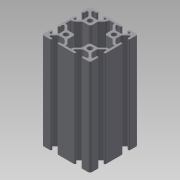
# Autodesk Inventor part: 25-5050
Saved by Autodesk Inventor 2013 (Build 170138000, 138)
## iProperties
Created: 2014-04-23
Part Number: 25-5050
Material: Generic
Document SubType Name: Modeling
Designer: Ross Bowman
Density: 1 g/cm^3
Engineer: Ross Bowman
Catalog Web Link: 8020.net
Vendor: 80/20 Inc.
Company: 80/20 Inc.
Author: Ross Bowman
Keywords: 80/20 , 8020 , T-Slot , Extrusion
Material: 6105-T5 Aluminum
Autodesk Inventor part; units mm, degrees
ref_plane "YZ Plane" through (0, 0, 0) normal (1, 0, 0) x (0, 1, 0)
ref_plane "XZ Plane" through (0, 0, 0) normal (0, 1, 0) x (-1, 0, 0)
ref_plane "XY Plane" through (0, 0, 0) normal (0, 0, 1) x (1, 0, 0)
sketch "Sketch1" plane through (0, 0, 0) normal (0, 0, 1) x (1, 0, 0)
  circle A0 centre (12.5, -12.5) radius 2.5
  circle A1 centre (12.5, 12.5) radius 2.5
  circle A2 centre (-12.5, 12.5) radius 2.5
  circle A3 centre (-12.5, -12.5) radius 2.5
  line L0 (-16.3975, 7.0892) -> (-19.6226, 3.8642)
  arc A4 (-14.8348, 7.7365) -> (-16.3975, 7.0892) centre (-14.8348, 5.5265) ccw
  line L1 (-9.6692, 7.7365) -> (-14.8348, 7.7365)
  arc A5 (-9.6692, 7.7365) -> (-7.4592, 9.9465) centre (-9.6692, 9.9465) ccw
  line L2 (-7.4592, 15.3582) -> (-7.4592, 9.9465)
  arc A6 (-6.8497, 16.6371) -> (-7.4592, 15.3582) centre (-5.3507, 15.138) ccw
  line L3 (-3.8502, 19.6366) -> (-6.8497, 16.6371)
  arc A7 (-3.8502, 19.6366) -> (-2.93, 21.8722) centre (-6.0718, 21.8582) ccw
  line L4 (-2.931, 22.0966) -> (-2.93, 21.8722)
  arc A8 (-2.171, 22.86) -> (-2.931, 22.0966) centre (-2.171, 22.1) ccw
  line L5 (2.171, 22.86) -> (-2.171, 22.86)
  arc A9 (2.931, 22.0966) -> (2.171, 22.86) centre (2.171, 22.1) ccw
  line L6 (2.93, 21.8722) -> (2.931, 22.0966)
  arc A10 (2.93, 21.8722) -> (3.8502, 19.6366) centre (6.0718, 21.8582) ccw
  line L7 (6.8497, 16.6371) -> (3.8502, 19.6366)
  arc A11 (7.4592, 15.3582) -> (6.8497, 16.6371) centre (5.3507, 15.138) ccw
  line L8 (7.4592, 9.9465) -> (7.4592, 15.3582)
  arc A12 (7.4592, 9.9465) -> (9.6692, 7.7365) centre (9.6692, 9.9465) ccw
  line L9 (14.8348, 7.7365) -> (9.6692, 7.7365)
  arc A13 (16.3975, 7.0892) -> (14.8348, 7.7365) centre (14.8348, 5.5265) ccw
  line L10 (19.6226, 3.8642) -> (16.3975, 7.0892)
  arc A14 (19.6226, 3.8642) -> (21.85, 2.9416) centre (21.85, 6.0916) ccw
  line L11 (22.1, 2.9496) -> (21.85, 2.9416)
  arc A15 (22.86, 2.1896) -> (22.1, 2.9496) centre (22.1, 2.1896) ccw
  line L12 (22.86, -2.1816) -> (22.86, 2.1896)
  arc A16 (22.1, -2.9416) -> (22.86, -2.1816) centre (22.1, -2.1816) ccw
  line L13 (21.85, -2.9416) -> (22.1, -2.9416)
  arc A17 (21.85, -2.9416) -> (19.6226, -3.8642) centre (21.85, -6.0916) ccw
  line L14 (16.3975, -7.0892) -> (19.6226, -3.8642)
  arc A18 (14.8348, -7.7365) -> (16.3975, -7.0892) centre (14.8348, -5.5265) ccw
  line L15 (9.6692, -7.7365) -> (14.8348, -7.7365)
  arc A19 (9.6692, -7.7365) -> (7.4592, -9.9465) centre (9.6692, -9.9465) ccw
  line L16 (7.4592, -15.3582) -> (7.4592, -9.9465)
  arc A20 (6.8497, -16.6371) -> (7.4592, -15.3582) centre (5.3507, -15.138) ccw
  line L17 (3.8502, -19.6366) -> (6.8497, -16.6371)
  arc A21 (3.8502, -19.6366) -> (2.93, -21.8722) centre (6.0718, -21.8582) ccw
  line L18 (2.931, -22.0966) -> (2.93, -21.8722)
  arc A22 (2.171, -22.86) -> (2.931, -22.0966) centre (2.171, -22.1) ccw
  line L19 (-2.171, -22.86) -> (2.171, -22.86)
  arc A23 (-2.931, -22.0966) -> (-2.171, -22.86) centre (-2.171, -22.1) ccw
  line L20 (-2.93, -21.8722) -> (-2.931, -22.0966)
  arc A24 (-2.93, -21.8722) -> (-3.8502, -19.6366) centre (-6.0718, -21.8582) ccw
  line L21 (-6.8497, -16.6371) -> (-3.8502, -19.6366)
  arc A25 (-7.4592, -15.3582) -> (-6.8497, -16.6371) centre (-5.3507, -15.138) ccw
  line L22 (-7.4592, -9.9465) -> (-7.4592, -15.3582)
  arc A26 (-7.4592, -9.9465) -> (-9.6692, -7.7365) centre (-9.6692, -9.9465) ccw
  line L23 (-14.8348, -7.7365) -> (-9.6692, -7.7365)
  arc A27 (-16.3975, -7.0892) -> (-14.8348, -7.7365) centre (-14.8348, -5.5265) ccw
  line L24 (-19.6226, -3.8642) -> (-16.3975, -7.0892)
  arc A28 (-19.6226, -3.8642) -> (-21.85, -2.9416) centre (-21.85, -6.0916) ccw
  line L25 (-22.1, -2.9416) -> (-21.85, -2.9416)
  arc A29 (-22.86, -2.1816) -> (-22.1, -2.9416) centre (-22.1, -2.1816) ccw
  line L26 (-22.86, 2.1896) -> (-22.86, -2.1816)
  arc A30 (-22.1, 2.9496) -> (-22.86, 2.1896) centre (-22.1, 2.1896) ccw
  line L27 (-21.85, 2.9416) -> (-22.1, 2.9496)
  arc A31 (-21.85, 2.9416) -> (-19.6226, 3.8642) centre (-21.85, 6.0916) ccw
  arc A32 (8.18, -25) -> (8.18, -22.86) centre (8.18, -23.93) ccw
  line L28 (8.18, -22.86) -> (6.0718, -22.86)
  arc A33 (5.3634, -21.1498) -> (6.0718, -22.86) centre (6.0718, -21.8582) ccw
  line L29 (5.3634, -21.1498) -> (8.5647, -17.9485)
  arc A34 (10.8063, -17.02) -> (8.5647, -17.9485) centre (10.8063, -20.19) ccw
  line L30 (10.8063, -17.02) -> (14.1937, -17.02)
  arc A35 (16.4353, -17.9485) -> (14.1937, -17.02) centre (14.1937, -20.19) ccw
  line L31 (16.4353, -17.9485) -> (19.6366, -21.1498)
  arc A36 (18.9282, -22.86) -> (19.6366, -21.1498) centre (18.9282, -21.8582) ccw
  line L32 (18.9282, -22.86) -> (16.82, -22.86)
  arc A37 (16.82, -22.86) -> (16.82, -25) centre (16.82, -23.93) ccw
  line L33 (16.82, -25) -> (23, -25)
  arc A38 (23, -25) -> (25, -23) centre (23, -23) ccw
  line L34 (25, -23) -> (25, -16.628)
  arc A39 (25, -16.628) -> (22.86, -16.628) centre (23.93, -16.628) ccw
  line L35 (22.86, -16.628) -> (22.86, -18.9112)
  arc A40 (21.1377, -19.6245) -> (22.86, -18.9112) centre (21.8511, -18.9112) ccw
  line L36 (21.1377, -19.6245) -> (17.9485, -16.4353)
  arc A41 (17.02, -14.1937) -> (17.9485, -16.4353) centre (20.19, -14.1937) ccw
  line L37 (17.02, -14.1937) -> (17.02, -10.8063)
  arc A42 (17.9485, -8.5647) -> (17.02, -10.8063) centre (20.19, -10.8063) ccw
  line L38 (17.9485, -8.5647) -> (21.1358, -5.3774)
  arc A43 (22.86, -6.0916) -> (21.1358, -5.3774) centre (21.85, -6.0916) ccw
  line L39 (22.86, -6.0916) -> (22.86, -8.372)
  arc A44 (22.86, -8.372) -> (25, -8.372) centre (23.93, -8.372) ccw
  line L40 (25, -8.372) -> (25, 8.18)
  arc A45 (25, 8.18) -> (22.86, 8.18) centre (23.93, 8.18) ccw
  line L41 (22.86, 8.18) -> (22.86, 6.0916)
  arc A46 (21.1358, 5.3774) -> (22.86, 6.0916) centre (21.85, 6.0916) ccw
  line L42 (21.1358, 5.3774) -> (17.9485, 8.5647)
  arc A47 (17.02, 10.8063) -> (17.9485, 8.5647) centre (20.19, 10.8063) ccw
  line L43 (17.02, 10.8063) -> (17.02, 14.1937)
  arc A48 (17.9485, 16.4353) -> (17.02, 14.1937) centre (20.19, 14.1937) ccw
  line L44 (17.9485, 16.4353) -> (21.1358, 19.6226)
  arc A49 (22.86, 18.9084) -> (21.1358, 19.6226) centre (21.85, 18.9084) ccw
  line L45 (22.86, 18.9084) -> (22.86, 16.82)
  arc A50 (22.86, 16.82) -> (25, 16.82) centre (23.93, 16.82) ccw
  line L46 (25, 16.82) -> (25, 23.1827)
  arc A51 (25, 23.1827) -> (23.0084, 25) centre (23.0084, 23) ccw
  line L47 (23.0084, 25) -> (16.82, 25)
  arc A52 (16.82, 25) -> (16.82, 22.86) centre (16.82, 23.93) ccw
  line L48 (16.82, 22.86) -> (18.9282, 22.86)
  arc A53 (19.6366, 21.1498) -> (18.9282, 22.86) centre (18.9282, 21.8582) ccw
  line L49 (19.6366, 21.1498) -> (16.4353, 17.9485)
  arc A54 (14.1937, 17.02) -> (16.4353, 17.9485) centre (14.1937, 20.19) ccw
  line L50 (14.1937, 17.02) -> (10.8063, 17.02)
  arc A55 (8.5647, 17.9485) -> (10.8063, 17.02) centre (10.8063, 20.19) ccw
  line L51 (8.5647, 17.9485) -> (5.3634, 21.1498)
  arc A56 (6.0718, 22.86) -> (5.3634, 21.1498) centre (6.0718, 21.8582) ccw
  line L52 (6.0718, 22.86) -> (8.18, 22.86)
  arc A57 (8.18, 22.86) -> (8.18, 25) centre (8.18, 23.93) ccw
  line L53 (8.18, 25) -> (-8.18, 25)
  arc A58 (-8.18, 25) -> (-8.18, 22.86) centre (-8.18, 23.93) ccw
  line L54 (-8.18, 22.86) -> (-6.0718, 22.86)
  arc A59 (-5.3634, 21.1498) -> (-6.0718, 22.86) centre (-6.0718, 21.8582) ccw
  line L55 (-5.3634, 21.1498) -> (-8.5647, 17.9485)
  arc A60 (-10.8063, 17.02) -> (-8.5647, 17.9485) centre (-10.8063, 20.19) ccw
  line L56 (-10.8063, 17.02) -> (-14.1937, 17.02)
  arc A61 (-16.4353, 17.9485) -> (-14.1937, 17.02) centre (-14.1937, 20.19) ccw
  line L57 (-16.4353, 17.9485) -> (-19.6366, 21.1498)
  arc A62 (-18.9282, 22.86) -> (-19.6366, 21.1498) centre (-18.9282, 21.8582) ccw
  line L58 (-18.9282, 22.86) -> (-16.82, 22.86)
  arc A63 (-16.82, 22.86) -> (-16.82, 25) centre (-16.82, 23.93) ccw
  line L59 (-16.82, 25) -> (-23.0084, 25)
  arc A64 (-23.0084, 25) -> (-25, 23.1827) centre (-23.0084, 23) ccw
  line L60 (-25, 23.1827) -> (-25, 16.82)
  arc A65 (-25, 16.82) -> (-22.86, 16.82) centre (-23.93, 16.82) ccw
  line L61 (-22.86, 16.82) -> (-22.86, 18.9084)
  arc A66 (-21.1358, 19.6226) -> (-22.86, 18.9084) centre (-21.85, 18.9084) ccw
  line L62 (-21.1358, 19.6226) -> (-17.9485, 16.4353)
  arc A67 (-17.02, 14.1937) -> (-17.9485, 16.4353) centre (-20.19, 14.1937) ccw
  line L63 (-17.02, 14.1937) -> (-17.02, 10.8063)
  arc A68 (-17.9485, 8.5647) -> (-17.02, 10.8063) centre (-20.19, 10.8063) ccw
  line L64 (-17.9485, 8.5647) -> (-21.1358, 5.3774)
  arc A69 (-22.86, 6.0916) -> (-21.1358, 5.3774) centre (-21.85, 6.0916) ccw
  line L65 (-22.86, 6.0916) -> (-22.86, 8.18)
  arc A70 (-22.86, 8.18) -> (-25, 8.18) centre (-23.93, 8.18) ccw
  line L66 (-25, 8.18) -> (-25, -8.372)
  arc A71 (-25, -8.372) -> (-22.86, -8.372) centre (-23.93, -8.372) ccw
  line L67 (-22.86, -8.372) -> (-22.86, -6.0916)
  arc A72 (-21.1358, -5.3774) -> (-22.86, -6.0916) centre (-21.85, -6.0916) ccw
  line L68 (-21.1358, -5.3774) -> (-17.9485, -8.5647)
  arc A73 (-17.02, -10.8063) -> (-17.9485, -8.5647) centre (-20.19, -10.8063) ccw
  line L69 (-17.02, -10.8063) -> (-17.02, -14.1937)
  arc A74 (-17.9485, -16.4353) -> (-17.02, -14.1937) centre (-20.19, -14.1937) ccw
  line L70 (-17.9485, -16.4353) -> (-21.1377, -19.6245)
  arc A75 (-22.86, -18.9112) -> (-21.1377, -19.6245) centre (-21.8511, -18.9112) ccw
  line L71 (-22.86, -18.9112) -> (-22.86, -16.628)
  arc A76 (-22.86, -16.628) -> (-25, -16.628) centre (-23.93, -16.628) ccw
  line L72 (-25, -16.628) -> (-25, -23)
  arc A77 (-25, -23) -> (-23, -25) centre (-23, -23) ccw
  line L73 (-23, -25) -> (-16.82, -25)
  arc A78 (-16.82, -25) -> (-16.82, -22.86) centre (-16.82, -23.93) ccw
  line L74 (-16.82, -22.86) -> (-18.9282, -22.86)
  arc A79 (-19.6366, -21.1498) -> (-18.9282, -22.86) centre (-18.9282, -21.8582) ccw
  line L75 (-19.6366, -21.1498) -> (-16.4353, -17.9485)
  arc A80 (-14.1937, -17.02) -> (-16.4353, -17.9485) centre (-14.1937, -20.19) ccw
  line L76 (-14.1937, -17.02) -> (-10.8063, -17.02)
  arc A81 (-8.5647, -17.9485) -> (-10.8063, -17.02) centre (-10.8063, -20.19) ccw
  line L77 (-8.5647, -17.9485) -> (-5.3634, -21.1498)
  arc A82 (-6.0718, -22.86) -> (-5.3634, -21.1498) centre (-6.0718, -21.8582) ccw
  line L78 (-6.0718, -22.86) -> (-8.18, -22.86)
  arc A83 (-8.18, -22.86) -> (-8.18, -25) centre (-8.18, -23.93) ccw
  line L79 (-8.18, -25) -> (8.18, -25)
  point P0 (0, 0)
  constraints: 160 end point, 160 point on circle, 84 centre point
extrude "Extrusion1" add sketch "Sketch1" against normal blind 100
body "Solid1"
